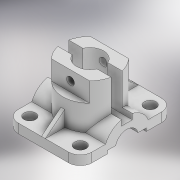
# Autodesk Inventor part: 组合体1
Saved by Autodesk Inventor 2020 (Build 240168000, 168)
## iProperties
Created: 2021-03-17
Part Number: 组合体1
Material: 常规
Document SubType Name: Modeling
Designer: Luorily
Density: 1 g/cm^3
Appearance: 默认
Author: Luorily
Autodesk Inventor part; units mm, degrees
ref_plane "YZ Plane" through (0, 0, 0) normal (1, 0, 0) x (0, 1, 0)
ref_plane "XZ Plane" through (0, 0, 0) normal (0, 1, 0) x (-1, 0, 0)
ref_plane "XY Plane" through (0, 0, 0) normal (0, 0, 1) x (1, 0, 0)
sketch "草图1" plane through (0, 0, 0) normal (1, 0, 0) x (0, 1, 0)
  line L0 (0, 0) -> (0, -120)
  line L1 (0, -120) -> (12, -120)
  line L2 (12, 0) -> (0, 0)
  arc A0 (12, -87.4955) -> (12, -32.5045) centre (0, -60) ccw
  line L3 (12, -120) -> (12, -87.4955)
  line L4 (12, -32.5045) -> (12, 0)
  point P0 (0, -89.9649)
  point P1 (0, -60)
  dimension "d0" = 120
  dimension "d1" = 12
  dimension "d2" = 60
  dimension "d67" = 12
  constraints: 10 end point, 5 perpendicular, 2 point on circle, 1 centre point, 1 coincident, 1 midpoint, 1 point on line, 1 vertical
  measures "d0" distance of L0.start L0.end
  measures "d1" distance of L0.end L1.end
  measures "d2" diameter of A0
  measures "d67" distance of L2.start L0.start
extrude "拉伸1" add sketch "草图1" along normal blind 95
sketch "草图3" plane through (0, 0, 0) normal (0, 1, 0) x (-1, 0, 0)
  circle A0 centre (-47.5, -60) radius 35
  point P0 (0, 0)
  dimension "d5" = 70
  constraints: 1 centre point
  measures "d5" diameter of A0
extrude "拉伸2" add sketch "草图3" along normal blind 70
sketch "草图4" plane through (47.5, 70, -60) normal (0, 1, 0) x (1, 0, 0)
  line L0 (47.5, -27.4955) -> (47.5, 27.4955) projected
  line L1 (47.5, -7) -> (-47.5, -7)
  line L2 (-47.5, -7) -> (-47.5, 7)
  line L3 (-47.5, -27.4955) -> (-47.5, 27.4955) projected
  line L4 (-47.5, 7) -> (47.5, 7)
  line L5 (47.5, 7) -> (47.5, -7)
  point P0 (-47.5, -60)
  point P1 (47.5, 7)
  dimension "d8" = 14
  constraints: 8 end point, 2 perpendicular, 2 point on line, 1 horizontal
  measures "d8" distance of L1.end L2.end
extrude "拉伸3" cut sketch "草图4" against normal blind 48
sketch "草图5" plane through (0, 70, 0) normal (0, 1, 0) x (1, 0, 0)
  arc A0 (13.2071, 53) -> (81.7929, 53) centre (47.5, 60) ccw projected
  line L0 (47.5, 35) -> (-14.0571, 35)
  line L1 (-14.0571, 35) -> (-14.0571, 7.8472)
  line L2 (-14.0571, 7.8472) -> (113.9638, 7.8472)
  line L3 (113.9638, 7.8472) -> (113.9638, 35)
  line L4 (113.9638, 35) -> (47.5, 35)
  line L5 (47.5, 85) -> (-16.5049, 85)
  line L6 (-16.5049, 85) -> (-16.5049, 106.9839)
  line L7 (-16.5049, 106.9839) -> (111.0264, 106.9839)
  line L8 (111.0264, 106.9839) -> (111.0264, 85)
  line L9 (111.0264, 85) -> (47.5, 85)
  point P0 (0, 0)
  dimension "d11" = 25
  dimension "d12" = 25
  constraints: 20 end point, 7 perpendicular, 2 point on line, 1 collinear
  measures "d11" distance of A0.centre L0.start
  measures "d12" distance of A0.centre L5.start
extrude "拉伸4" cut sketch "草图5" against normal blind 25
sketch "草图6" plane through (71.9949, 70, -85) normal (0, 0, -1) x (-1, 0, 0)
  line L0 (0, -25) -> (48.9898, -25) projected
  circle A0 centre (24.4949, -12.5) radius 5
  point P0 (71.9949, -70)
  dimension "d15" = 10
  constraints: 1 centre point
  measures "d15" diameter of A0
hole "孔1" at (47.5, 57.5, -85) direction (0, 0, 1) diameter 10 end through all
sketch "草图7" plane through (95, 0, 0) normal (1, 0, 0) x (0, 0, -1)
  line L0 (0, 0) -> (120, 0) projected
  line L1 (0, 0) -> (120, 0) projected
  arc A0 (74.4568, 4) -> (45.5432, 4) centre (60, 0) ccw
  line L2 (60, 0) -> (35, 0)
  line L3 (35, 0) -> (35, 4)
  line L4 (85, 4) -> (85, 0)
  line L5 (35, 4) -> (45.5432, 4)
  line L6 (74.4568, 4) -> (85, 4)
  line L7 (60, 0) -> (85, 0)
  dimension "d23" = 30
  dimension "d24" = 25
  dimension "d25" = 4
  dimension "d26" = 50
  constraints: 12 end point, 4 perpendicular, 2 point on circle, 2 point on line, 1 centre point, 1 collinear, 1 midpoint
  measures "d23" diameter of A0
  measures "d24" distance of L2.start L2.end
  measures "d25" distance of L2.end L3.end
  measures "d26" distance of L3.end L4.start
extrude "拉伸5" cut sketch "草图7" against normal blind 100
fillet "圆角1" radius 15 1 edges at (0, 6, -120)
fillet "圆角2" radius 15 3 edges at (95, 6, -120) (95, 6, 0) (0, 6, 0)
sketch "草图9" plane through (47.5, 12, -60) normal (0, 1, 0) x (1, 0, 0)
  arc A0 (-47.5, -45) -> (-32.5, -60) centre (-32.5, -45) ccw projected
  arc A1 (32.5, -60) -> (47.5, -45) centre (32.5, -45) ccw projected
  point P0 (-47.5, -60)
  point P1 (-32.5, -45)
  point P2 (32.5, -45)
  constraints: 2 coincident
hole "孔2" at (15, 12, -15) at (80, 12, -15) direction (0, -1, 0) diameter 15 end through all
sketch "草图10" plane through (47.5, 12, -60) normal (0, 1, 0) x (1, 0, 0)
  arc A0 (47.5, 45) -> (32.5, 60) centre (32.5, 45) ccw projected
  arc A1 (-32.5, 60) -> (-47.5, 45) centre (-32.5, 45) ccw projected
  point P0 (-47.5, -60)
  constraints: 2 coincident
hole "孔3" at (15, 12, -105) at (80, 12, -105) direction (0, -1, 0) diameter 15 end through all
ref_plane "工作平面2" through (47.5, 12, -120) normal (-1, 0, 0) x (0, 0, 1)
sketch "草图11" plane through (47.5, 12, -120) normal (-1, 0, 0) x (0, 0, 1)
  line L0 (0, 0) -> (0, -12) projected
  line L1 (25, 0) -> (25, 33) projected
  line L2 (15, 0) -> (32.5045, 0) projected
  line L3 (0, 0) -> (25, 20)
  line L4 (25, 20) -> (25, -12)
  line L5 (35, -12) -> (15, -12) projected
  line L6 (120, -12) -> (120, 0) projected
  line L7 (120, 0) -> (95, 20)
  line L8 (95, 0) -> (95, 33) projected
  line L9 (95, 20) -> (95, -5.625)
  dimension "d46" = 20
  dimension "d53" = 20
  constraints: 8 end point, 2 point on line, 1 midpoint, 1 vertical
  measures "d46" vertical distance of L0.start L3.end
  measures "d53" vertical distance of L6.end L7.end
extrude "加强筋1" add sketch "草图11" along normal mid plane 5 rib yes fills toward (0.05, -6) open curves L0 L3 L4
extrude "加强筋2" add sketch "草图11" along normal mid plane 5 rib yes fills toward (119.95, -6) open curves L6 L7 L9
sketch "草图12" plane through (0, 70, 0) normal (0, 1, 0) x (1, 0, 0)
  arc A0 (81.7929, 67) -> (71.9949, 85) centre (47.5, 60) ccw projected
  point P0 (0, 0)
  constraints: 1 coincident
hole "孔4" at (47.5, 70, -60) direction (0, -1, 0) diameter 35 end through all
equation "\"d67\" = d1"
